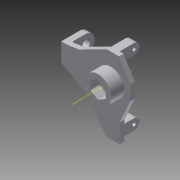
# Autodesk Inventor part: servo_gimbal_interpart_1
Saved by Autodesk Inventor 2015 SP1 (Build 190203100, 203)
## iProperties
Created: 2015-07-15
Part Number: servo_gimbal_interpart_1
Material: ABS Plastic
Document SubType Name: Modeling
Designer: Alexandre Cherpillod
Density: 1.06 g/cm^3
Appearance: Smooth - White
Mass: 2.09818 g
Surface Area: 21.8206 cm^2
Volume: 1.97941 cm^3
Author: Alexandre Cherpillod
Autodesk Inventor part; units mm, degrees
ref_plane "YZ Plane" through (0, 0, 0) normal (1, 0, 0) x (0, 1, 0)
ref_plane "XZ Plane" through (0, 0, 0) normal (0, 1, 0) x (-1, 0, 0)
ref_plane "XY Plane" through (0, 0, 0) normal (0, 0, 1) x (1, 0, 0)
sketch "Sketch2" plane through (0, 0, 0) normal (0, 1, 0) x (-1, 0, 0)
  line L0 (2.5334, 16.1644) -> (0.0334, 16.1644)
  line L1 (0.0334, 16.1644) -> (0.0334, 24.1644)
  line L2 (0.0334, 24.1644) -> (2.5334, 24.1644)
  line L3 (2.5334, 24.1644) -> (2.5334, 16.1644)
  line L4 (-20.5666, -1.6356) -> (-16.9666, -1.6356)
  line L5 (-16.9666, -1.6356) -> (-16.9666, 2.9644)
  line L6 (-16.9666, 2.9644) -> (-20.5666, 2.9644)
  line L7 (-20.5666, 2.9644) -> (-20.5666, -1.6356)
  line L8 (-20.5666, 30.9644) -> (-16.9666, 30.9644)
  line L9 (-16.9666, 30.9644) -> (-16.9666, 26.3644)
  line L10 (-16.9666, 26.3644) -> (-20.5666, 26.3644)
  line L11 (-20.5666, 26.3644) -> (-20.5666, 30.9644)
  point P0 (0, 0)
  point P1 (-20.5666, 0.6644)
  point P2 (-20.5666, 28.6644)
  point P3 (0.0334, 20.1644)
  dimension "d4" = 4.6
  dimension "d5" = 3.6
  dimension "d6" = 2.5
  dimension "d7" = 8
  dimension "d8" = 28
  dimension "d9" = 8.5
  dimension "d59" = 20.6
  constraints: 25 end point, 7 parallel, 3 midpoint, 3 perpendicular, 2 point on line, 1 collinear, 1 horizontal
  measures "d4" distance of L10.end L8.start
  measures "d5" distance of L9.end L10.end
  measures "d6" distance of L1.end L2.end
  measures "d7" distance of L2.end L0.start
  measures "d8" distance of point (-20.567, 0.664) point (-20.567, 28.664)
  measures "d9" vertical distance of point (-20.567, 28.664) point (0.033, 20.164)
  measures "d59" distance between parallel lines of L1 L11
extrude "Extrusion2" add sketch "Sketch2" along normal blind 8.5
sketch "Sketch3" plane through (0, 8.5, 0) normal (0, 1, 0) x (1, 0, 0)
  line L0 (-2.5334, -24.1644) -> (-0.0334, -24.1644)
  line L1 (-0.0334, -24.1644) -> (-0.0334, -16.1644)
  line L2 (-0.0334, -16.1644) -> (-2.5334, -16.1644)
  line L3 (-2.5334, -16.1644) -> (-2.5334, -24.1644)
  point P0 (0, 0)
  constraints: 8 end point, 2 parallel, 1 horizontal, 1 perpendicular
extrude "Extrusion3" add sketch "Sketch3" along normal blind 1.4
fillet "Fillet1" radius 2.3 4 edges at (18.7666, 8.5, 30.9644) (18.7666, 8.5, 26.3644) (18.7666, 8.5, 2.9644) (18.7666, 8.5, -1.6356)
fillet "Fillet2" radius 4 2 edges at (-1.2834, 9.9, 24.1644) (-1.2834, 9.9, 16.1644)
sketch "Sketch4" plane through (-0.0334, 0, 24.1644) normal (1, 0, 0) x (0, 0, -1)
  line L0 (8, 0) -> (0, 0) projected
  line L1 (4, 0) -> (4, 9.2517) construction
  line L2 (-6.8, 0) -> (-2.2, 0) construction
  line L3 (25.8, 0) -> (21.2, 0) construction
  line L4 (-4.5, 0) -> (-4.5, 8.5) construction
  arc A0 (-2.2, 6.2) -> (-6.8, 6.2) centre (-4.5, 6.2) ccw construction
  line L5 (23.5, 0) -> (23.5, 8.5) construction
  circle A1 centre (4, 6.3) radius 1.75
  circle A2 centre (23.5, 6.3) radius 0.75
  circle A3 centre (-4.5, 6.3) radius 0.75
  point P0 (24.1644, 0)
  dimension "d17" = 3.5
  dimension "d19" = 1.5
  dimension "d20" = 1.5
  dimension "d21" = 6.3
  dimension "d22" = 6.3
  dimension "d23" = 6.3
  constraints: 6 end point, 3 centre point, 3 midpoint, 3 point on line, 3 vertical, 1 point on circle
  measures "d17" diameter of A1
  measures "d19" diameter of A2
  measures "d20" diameter of A3
  measures "d21" distance from line of L2 A3.centre
  measures "d22" distance from line of L3 A2.centre
  measures "d23" distance from line of L0 A1.centre
extrude "Extrusion4" cut sketch "Sketch4" along normal through all both and the other way through all
sketch "Sketch5" plane through (0, 0, 0) normal (0, -1, 0) x (1, 0, 0)
  line L0 (-2.5334, 16.1644) -> (6.8584, 11.1365)
  line L1 (6.8584, 11.1365) -> (16.9666, -1.6356)
  line L2 (16.9666, -1.6356) -> (20.5666, -1.6356)
  line L3 (20.5666, -1.6356) -> (16.9666, -1.6356) projected
  line L4 (20.5666, -1.6356) -> (22.5666, -1.6356)
  line L5 (22.2666, 30.9644) -> (20.5666, 30.9644)
  line L6 (20.5666, 30.9644) -> (16.9666, 30.9644)
  line L7 (16.9666, 30.9644) -> (5.172, 24.9376)
  line L8 (5.172, 24.9376) -> (-0.0334, 24.1644)
  line L9 (-0.0334, 24.1644) -> (-2.5334, 24.1644)
  line L10 (-0.0334, 24.1644) -> (-2.5334, 24.1644) projected
  line L11 (-2.5334, 24.1644) -> (-2.5334, 16.1644)
  line L12 (22.2666, 30.9644) -> (27.1025, 22.846)
  line L13 (27.1025, 22.846) -> (27.1025, 16.6045)
  line L14 (27.1025, 16.6045) -> (22.5666, 6.5187)
  line L15 (22.5666, 6.5187) -> (22.5666, -1.6356)
  point P0 (0, 0)
  dimension "d26" = 2
  constraints: 28 end point, 3 equal length, 2 perpendicular, 1 collinear, 1 point on line, 1 vertical
  measures "d26" distance of L2.end L4.end
extrude "Extrusion5" add sketch "Sketch5" along normal blind 2
sketch "Sketch7" plane through (0, -2, 0) normal (0, -1, 0) x (1, 0, 0)
  line L0 (16.9666, 2.9644) -> (20.5666, 2.9644) projected
  line L1 (18.7666, 2.9644) -> (18.7666, 26.3644) construction
  line L2 (20.5666, 26.3644) -> (16.9666, 26.3644) projected
  line L3 (18.7666, 15.8122) -> (15.4666, 17.7174)
  line L4 (15.4666, 17.7174) -> (15.4666, 21.5279)
  line L5 (15.4666, 21.5279) -> (18.7666, 23.4332)
  line L6 (18.7666, 23.4332) -> (22.0666, 21.5279)
  line L7 (22.0666, 21.5279) -> (22.0666, 17.7174)
  line L8 (22.0666, 17.7174) -> (18.7666, 15.8122)
  line L9 (20.5666, 29.4144) -> (20.5666, 27.9144) construction
  line L10 (20.5666, 29.5605) -> (16.9666, 27.9144) construction
  line L11 (16.9666, 27.9144) -> (16.9666, 29.4144) construction
  line L12 (20.5666, 26.7294) -> (15.111, 29.4144) construction
  line L13 (16.9666, 29.4144) -> (20.5666, 29.4144) construction
  circle A0 centre (18.7666, 19.6227) radius 5.75
  point P0 (0, 0)
  point P1 (17.8388, 28.0719)
  dimension "d29" = 8.5
  dimension "d30" = 6.6
  dimension "d31" = 11.5
  constraints: 19 end point, 5 point on line, 3 midpoint, 1 centre point, 1 coincident, 13 other
  measures "d29" distance of point (17.839, 28.072) point (18.767, 19.623)
  measures "d30" distance between parallel lines of L7 L4
  measures "d31" diameter of A0
extrude "Extrusion6" add sketch "Sketch7" along normal blind 5.5
chamfer "Chamfer1" distance 0.5 angle 45 1 edges at (-0.0334, 0, 20.1644)
hole "Hole1" at (18.7666, 0, 19.6227) direction (0, -1, 0) diameter 2.4 end through all
hole "Hole2" at (18.7666, 0, 19.6227) direction (0, -1, 0) diameter 4.6 depth 1.7
sketch "Sketch8" plane through (0, -2, 0) normal (0, -1, 0) x (1, 0, 0)
  line L0 (18.7666, 23.4332) -> (22.0666, 21.5279)
  line L1 (22.0666, 21.5279) -> (22.0666, 17.7174)
  line L2 (22.0666, 17.7174) -> (18.7666, 15.8122)
  line L3 (18.7666, 15.8122) -> (15.4666, 17.7174)
  line L4 (15.4666, 17.7174) -> (15.4666, 21.5279)
  line L5 (15.4666, 21.5279) -> (18.7666, 23.4332)
  circle A0 centre (18.7666, 19.6227) radius 1.2
  point P0 (0, 0)
  constraints: 12 end point, 2 coincident, 1 centre point, 13 other
extrude "Extrusion7" add sketch "Sketch8" along normal blind 1.5
body "Solid2"
